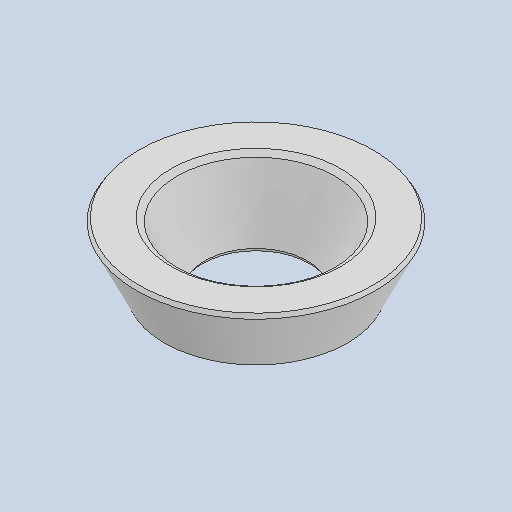
# Autodesk Inventor part: Washer
Saved by Autodesk Inventor 2023 (Build 270158000, 158)
## iProperties
Created: 2023-08-22
Part Number: Washer
Material: Generic
Document SubType Name: Modeling
Designer: chriboehm
Density: 1 g/cm^3
Appearance: Default
Mass: 0.173284 g
Surface Area: 2.86595 cm^2
Volume: 0.173284 cm^3
Author: chriboehm
Autodesk Inventor part; units mm, degrees
ref_plane "YZ Plane" through (0, 0, 0) normal (1, 0, 0) x (0, 1, 0)
ref_plane "XZ Plane" through (0, 0, 0) normal (0, 1, 0) x (-1, 0, 0)
ref_plane "XY Plane" through (0, 0, 0) normal (0, 0, 1) x (1, 0, 0)
sketch "Sketch1" plane through (0, 0, 0) normal (0, 0, 1) x (1, 0, 0)
  line L0 (0, 0) -> (0, 3.3)
  line L1 (2.45, 0) -> (4.45, 0)
  line L2 (4.45, 0) -> (6, 3.3)
  line L3 (6, 3.3) -> (4, 3.3)
  line L4 (4, 3.3) -> (2.45, 0)
  point P0 (3.45, 0)
  point P1 (5, 3.3)
  dimension "d1" = 3.3
  dimension "d3" = 2
  dimension "d5" = 8
  dimension "d6" = 4.9
  constraints: 10 end point, 2 midpoint, 2 parallel, 1 horizontal, 1 point on line, 1 vertical
  measures "d1" distance from line of point (5, 3.3) L1
  measures "d3" distance of L2.end L3.end
  measures "d5" diameter of L3.end L0
  measures "d6" diameter of L1.start L0
revolve "Revolution1" add sketch "Sketch1" angle 360 about axis through (0, 0, 0) along (0, 1, 0)
chamfer "Chamfer1" distance 0.2 angle 45 4 edges at (-6, 3.3, 0) (-4.45, 0, 0) (-4, 3.3, 0) (-2.45, 0, 0)
body "Solid1"
